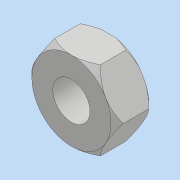
# Autodesk Inventor part: Bolt
Saved by Autodesk Inventor 2018 (Build 220112000, 112)
## iProperties
Created: 2020-08-11
Part Number: Bolt
Material: Generic
Document SubType Name: Modeling
Designer: ASUS
Density: 1 g/cm^3
Appearance: Default
Author: ASUS
Autodesk Inventor part; units mm, degrees
ref_plane "YZ Plane" through (0, 0, 0) normal (1, 0, 0) x (0, 1, 0)
ref_plane "XZ Plane" through (0, 0, 0) normal (0, 1, 0) x (-1, 0, 0)
ref_plane "XY Plane" through (0, 0, 0) normal (0, 0, 1) x (1, 0, 0)
sketch "Sketch3" plane through (0, 0, 0) normal (0, 1, 0) x (-1, 0, 0)
  line L0 (-4.9048, -8.5016) -> (-9.815, -0.0031)
  line L1 (-9.815, -0.0031) -> (-4.9102, 8.4984)
  line L2 (-4.9102, 8.4984) -> (4.9048, 8.5016)
  line L3 (4.9048, 8.5016) -> (9.815, 0.0031)
  line L4 (9.815, 0.0031) -> (4.9102, -8.4984)
  line L5 (4.9102, -8.4984) -> (-4.9048, -8.5016)
  point P0 (0, 0)
  point P1 (0, 0)
  dimension "d1" = 17
  constraints: 12 end point, 1 coincident, 13 other
  measures "d1" distance between parallel lines of L2 L5
extrude "Extrusion1" add sketch "Sketch3" along normal blind 8
sketch "Sketch4" plane through (0, 8, 0) normal (0, 1, 0) x (1, 0, 0)
  circle A0 centre (0, 0) radius 8.6061
  constraints: 1 centre point, 1 coincident
extrude "Extrusion2" cut sketch "Sketch4" against normal through all draft 45 keep common part
sketch "Sketch22" plane through (0, 0, 0) normal (0, -1, 0) x (1, 0, 0)
  circle A0 centre (0, 0) radius 8.5
  line L0 (6.6894, 5.4144) -> (8.0357, 3.0809) projected
  constraints: 1 centre point, 1 coincident, 1 tangent
extrude "Extrusion12" cut sketch "Sketch22" against normal blind 8 draft 45 keep common part
sketch "Sketch23" plane through (0, 0, 0) normal (0, -1, 0) x (1, 0, 0)
  circle A0 centre (0, 0) radius 4
  dimension "d111" = 8
  constraints: 1 centre point, 1 coincident
  measures "d111" diameter of A0
extrude "Extrusion13" cut sketch "Sketch23" against normal blind 8
body "Solid1"
